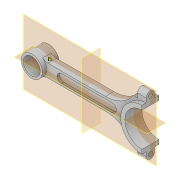
# Autodesk Inventor part: 7.3_Connecting_Rod
Saved by Autodesk Inventor 2017 (Build 210142000, 142)
## iProperties
Created: 2018-11-02
Part Number: 7.3_Connecting_Rod
Material: Generic
Document SubType Name: Modeling
Designer: jpb34
Density: 1 g/cm^3
Appearance: Default
Mass: 51.7401 g
Surface Area: 217.298 cm^2
Volume: 51.7401 cm^3
Author: jpb34
Autodesk Inventor part; units mm, degrees
sketch "Sketch1" plane through (0, 0, 0) normal (0, 0, 1) x (1, 0, 0)
  circle A0 centre (-76.2, 0) radius 15.875
  line L0 (-38.1, 0) -> (38.1, 0) construction
  line L1 (-38.1, -6.35) -> (38.1, -6.35)
  line L2 (38.1, 6.35) -> (-38.1, 6.35)
  arc A1 (-38.1, 6.35) -> (-38.1, -6.35) centre (-38.1, 0) ccw
  arc A2 (38.1, -6.35) -> (38.1, 6.35) centre (38.1, 0) ccw
  arc A3 (88.9, 31.75) -> (88.9, -31.75) centre (88.9, 0) ccw
  circle A4 centre (-76.2, 0) radius 12.7
  arc A5 (88.9, 25.4) -> (88.9, -25.4) centre (88.9, 0) ccw
  line L3 (88.9, 31.75) -> (88.9, 25.4)
  line L4 (88.9, -25.4) -> (88.9, -31.75)
  line L5 (88.9, 31.75) -> (69.85, 31.75)
  line L6 (88.9, -31.75) -> (69.85, -31.75)
  line L7 (-58.2395, 9.525) -> (27.8487, 9.525)
  line L8 (-58.2395, -9.525) -> (27.8487, -9.525)
  arc A6 (27.8487, 9.525) -> (69.85, 31.75) centre (27.8487, 60.325) ccw
  arc A7 (69.85, -31.75) -> (27.8487, -9.525) centre (27.8487, -60.325) ccw
  arc A8 (-66.2219, 12.3472) -> (-58.2395, 9.525) centre (-58.2395, 22.225) ccw
  arc A9 (-58.2395, -9.525) -> (-66.2219, -12.3472) centre (-58.2395, -22.225) ccw
  point P0 (0, 0)
  point P1 (0, 0)
  dimension "d0" = 31.75
  dimension "d1" = 25.4
  dimension "d2" = 12.7
  dimension "d3" = 76.2
  dimension "d4" = 165.1
  dimension "d5" = 50.8
  dimension "d6" = 63.5
  dimension "d7" = 50.8
  dimension "d8" = 19.05
  dimension "d9" = 19.05
  dimension "d12" = 19.05
  dimension "d13" = 9.525
  dimension "d15" = 101.6
  dimension "d16" = 101.6
  dimension "d18" = 25.4
  dimension "d19" = 0
  dimension "d39" = 31.75
  dimension "d41" = 25.4
  constraints: 20 end point, 18 point on circle, 12 tangent, 10 centre point, 4 horizontal, 3 coincident, 2 parallel, 2 vertical, 1 midpoint
  measures "d0" diameter of A0
  measures "d1" diameter of A4
  measures "d2" distance between parallel lines of L2 L1
  measures "d3" distance of L2.start L2.end
  measures "d4" distance of A3.centre A0.centre
  measures "d5" horizontal distance of A3.centre L2.start
  measures "d6" diameter of A3
  measures "d7" diameter of A5
  measures "d8" distance of L3.start L5.end
  measures "d9" distance of L4.end L6.end
  measures "d12" distance between parallel lines of L8 L7
  measures "d13" distance from line of L7 point (0, 0)
  measures "d15" diameter of A6
  measures "d16" diameter of A7
  measures "d18" diameter of A8
  measures "d19" vertical distance of A0.centre point (0, 0)
  measures "d39" distance between parallel lines of L5 L0
  measures "d41" diameter of A9
extrude "Base" add sketch "Sketch1" along normal mid plane 12.7
extrude "Indent" add sketch "Sketch1" along normal mid plane 6.35 contours A1 L2 A2 L1
extrude "Extrusion4" add sketch "Sketch1" along normal mid plane 25.4 contours L3 A5 L4 A3
sketch "Sketch3" plane through (88.9, 25.4, 12.7) normal (1, 0, 0) x (0, 0, -1)
  line L0 (6.35, 6.35) -> (19.05, 6.35)
  line L1 (19.05, 6.35) -> (19.05, 12.7)
  line L2 (6.35, 12.7) -> (6.35, 6.35)
  line L3 (6.35, 6.35) -> (19.05, 6.35) projected
  line L4 (0, 0) -> (0, 6.35) projected
  line L5 (25.4, 0) -> (0, 0) projected
  line L6 (25.4, 6.35) -> (25.4, 0) projected
  arc A0 (19.05, 12.7) -> (6.35, 12.7) centre (12.7, 12.7) ccw
  circle A1 centre (12.7, 12.7) radius 3.175
  line L7 (-5.08, -25.4) -> (30.48, -25.4) projected
  line L8 (6.35, -57.15) -> (19.05, -57.15)
  line L9 (19.05, -57.15) -> (19.05, -63.5)
  line L10 (6.35, -63.5) -> (6.35, -57.15)
  line L11 (6.35, -57.15) -> (19.05, -57.15)
  line L12 (6.35, -57.15) -> (19.05, -57.15)
  arc A2 (6.35, -63.5) -> (19.05, -63.5) centre (12.7, -63.5) ccw
  circle A3 centre (12.7, -63.5) radius 3.175
  line L13 (6.35, 6.35) -> (19.05, 6.35) projected
  line L14 (19.05, 6.35) -> (25.4, 6.35) projected
  line L15 (0, 6.35) -> (6.35, 6.35) projected
  point P0 (12.7, -25.4)
  dimension "d28" = 0
  dimension "d30" = 12.7
  dimension "d31" = 6.35
  dimension "d32" = 6.35
  dimension "d42" = 6.35
  dimension "d43" = 76.2
  dimension "d44" = 6.35
  constraints: 16 end point, 8 symmetric about line, 4 centre point, 4 point on circle, 2 coincident, 1 horizontal, 1 parallel, 1 perpendicular, 2 other
  measures "d28" distance between parallel lines of L3 L0
  measures "d30" distance between parallel lines of L2 L1
  measures "d31" distance between parallel lines of L2 L4
  measures "d32" diameter of A1
  measures "d42" radius of A0
  measures "d43" distance of A2.centre A0.centre
  measures "d44" distance of L0.end L1.end
extrude "Extrusion5" add sketch "Sketch3" against normal blind 12.7 contours L2 A0 L1 L0 | L8 L9 A2 L10
sketch "Sketch4" plane through (0, 0, 6.35) normal (0, 0, 1) x (1, 0, 0)
  arc A0 (-66.2219, 12.3472) -> (-66.2219, -12.3472) centre (-76.2, 0) ccw projected
  circle A1 centre (-76.2, 0) radius 12.7 projected
  circle A2 centre (-76.2, 0) radius 12.7
  circle A3 centre (-76.2, 0) radius 15.875
  arc A4 (88.9, 31.75) -> (88.9, -31.75) centre (88.9, 0) ccw projected
  line L0 (88.9, 38.1) -> (88.9, 31.75) projected
  line L1 (88.9, 38.1) -> (76.2, 38.1) projected
  line L2 (76.2, 31.75) -> (76.2, 38.1) projected
  line L3 (76.2, 31.75) -> (69.85, 31.75) projected
  arc A5 (27.8487, 9.525) -> (69.85, 31.75) centre (27.8487, 60.325) ccw projected
  line L4 (27.8487, 9.525) -> (-58.2395, 9.525) projected
  arc A6 (-66.2219, 12.3472) -> (-58.2395, 9.525) centre (-58.2395, 22.225) ccw projected
  arc A7 (-58.2395, -9.525) -> (-66.2219, -12.3472) centre (-58.2395, -22.225) ccw projected
  line L5 (-58.2395, -9.525) -> (27.8487, -9.525) projected
  arc A8 (69.85, -31.75) -> (27.8487, -9.525) centre (27.8487, -60.325) ccw projected
  line L6 (69.85, -31.75) -> (76.2, -31.75) projected
  line L7 (76.2, -38.1) -> (76.2, -31.75) projected
  line L8 (88.9, -38.1) -> (76.2, -38.1) projected
  line L9 (88.9, -31.75) -> (88.9, -38.1) projected
  point P0 (0, 0)
  constraints: 2 centre point, 2 coincident
extrude "Extrusion6" add sketch "Sketch4" against normal blind 19.05 and the other way blind 6.35 contours A3 A0
body "Solid1"
